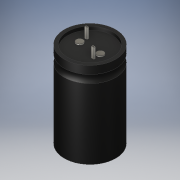
# Autodesk Inventor part: capacitor (LGN2X151MELB50)
Saved by Autodesk Inventor 2017 (Build 210142000, 142)
## iProperties
Part Number: capacitor (LGN2X151MELB50)
Material: Generisch
Document SubType Name: Modeling
Designer: ExCISS
Density: 1 g/cm^3
Appearance: Glänzend - schwarz
Author: ExCISS
Autodesk Inventor part; units mm, degrees
ref_plane "YZ Plane" through (0, 0, 0) normal (1, 0, 0) x (0, 1, 0)
ref_plane "XZ Plane" through (0, 0, 0) normal (0, 1, 0) x (-1, 0, 0)
sketch "Skizze1" plane through (0, 0, 0) normal (0, 1, 0) x (-1, 0, 0)
  line L0 (0, 0) -> (0, 50)
  line L1 (0, 50) -> (-15, 50)
  line L2 (-15, 50) -> (-15, 45.4)
  line L3 (-15, 40.8) -> (-15, 0)
  arc A0 (-15, 40.8) -> (-15, 45.4) centre (-20.6528, 43.1) ccw
  line L4 (0, 0) -> (-15, 0)
  line L5 (0, -10) -> (0, 60) projected
  dimension "d0" = 50
  dimension "d1" = 15
  dimension "d2" = 4.6
  dimension "d72" = 14.55
  dimension "d73" = 4.6
  constraints: 10 end point, 2 perpendicular, 2 point on circle, 2 point on line, 1 centre point, 1 horizontal, 1 vertical
  measures "d0" distance of L0.start L0.end
  measures "d1" distance of L0.end L1.end
  measures "d2" distance of L1.end L2.end
  measures "d72" distance edge to line of A0 L0
  measures "d73" distance of L2.end L3.start
revolve "Umdrehung1" add sketch "Skizze1" angle 360 about axis through (0, 0, -10) along (0, 0, 1)
sketch "Skizze3" plane through (0, 0, 50) normal (0, 0, 1) x (1, 0, 0)
  circle A0 centre (0, 0) radius 13.05
  dimension "d10" = 26.1
  constraints: 1 centre point, 1 coincident
  measures "d10" diameter of A0
extrude "Extrusion2" cut sketch "Skizze3" against normal blind 2
sketch "Skizze7" plane through (0, 0, 0) normal (0, 0, -1) x (-1, 0, 0)
  circle A0 centre (0, 0) radius 12.8
  dimension "d19" = 25.6
  constraints: 1 centre point, 1 coincident
  measures "d19" diameter of A0
extrude "Extrusion4" cut sketch "Skizze7" against normal blind 0.02
sketch "Skizze17" plane through (0, 0, 48) normal (0, 0, 1) x (1, 0, 0)
  line L0 (-4.2414, 0) -> (6, 0) construction
  line L1 (6, 0) -> (-6, 0) construction
  line L2 (6, 0) -> (6, -3.5) construction
  line L3 (-6, 0) -> (-6, 3.5) construction
  line L4 (-6, 3.5) -> (6, -3.5) construction
  circle A0 centre (-6, 0) radius 2
  circle A1 centre (6, 0) radius 2
  line L5 (-6.75, 4.5) -> (-5.25, 4.5)
  line L6 (-5.25, 4.5) -> (-5.25, 3.5)
  line L7 (-5.25, 3.5) -> (-6.75, 3.5)
  line L8 (-6.75, 3.5) -> (-6.75, 4.5)
  line L9 (6.75, -3.5) -> (5.25, -3.5)
  line L10 (5.25, -3.5) -> (5.25, -4.5)
  line L11 (5.25, -4.5) -> (6.75, -4.5)
  line L12 (6.75, -4.5) -> (6.75, -3.5)
  point P0 (0, 0)
  point P1 (0, 0)
  dimension "d54" = 12
  dimension "d55" = 3.5
  dimension "d56" = 3.5
  dimension "d57" = 4
  dimension "d58" = 4
  dimension "d59" = 1.5
  dimension "d60" = 1
  dimension "d61" = 1.5
  dimension "d62" = 1
  constraints: 26 end point, 4 parallel, 3 coincident, 3 horizontal, 3 midpoint, 2 centre point, 2 perpendicular, 2 vertical, 1 point on line
  measures "d54" distance of L0.end L1.end
  measures "d55" distance of L2.end L0.end
  measures "d56" distance of L3.end L1.end
  measures "d57" diameter of A0
  measures "d58" diameter of A1
  measures "d59" distance of L6.end L7.end
  measures "d60" distance of L5.end L6.end
  measures "d61" distance of L11.end L10.end
  measures "d62" distance of L10.end L9.end
extrude "Extrusion8" add sketch "Skizze17" along normal blind 0.6 contours A0 | A1
sketch "Skizze18" plane through (0, 0, 48) normal (0, 0, 1) x (1, 0, 0)
  line L0 (-6.75, 4.5) -> (-5.25, 4.5)
  line L1 (-5.25, 4.5) -> (-5.25, 3.5)
  line L2 (-5.25, 3.5) -> (-6.75, 3.5)
  line L3 (-6.75, 3.5) -> (-6.75, 4.5)
  line L4 (6.75, -3.5) -> (5.25, -3.5)
  line L5 (5.25, -3.5) -> (5.25, -4.5)
  line L6 (5.25, -4.5) -> (6.75, -4.5)
  line L7 (6.75, -4.5) -> (6.75, -3.5)
  point P0 (0, 0)
  point P1 (-6, 3.5)
  point P2 (6, -3.5)
  dimension "d66" = 1.5
  dimension "d67" = 1
  dimension "d68" = 1.5
  dimension "d69" = 1
  constraints: 16 end point, 4 parallel, 2 horizontal, 2 midpoint, 2 perpendicular
  measures "d66" distance of L1.end L2.end
  measures "d67" distance of L1.start L1.end
  measures "d68" distance of L6.end L5.end
  measures "d69" distance of L5.end L4.end
extrude "Extrusion9" add sketch "Skizze18" along normal blind 6
sketch "Skizze9" plane through (0, 0, 0.02) normal (0, 0, -1) x (-1, 0, 0)
  line L0 (-7.5, 0) -> (7.5, 0) construction
  line L1 (0, 4.0384) -> (0, 7.5) construction
  line L2 (0, 7.5) -> (0, -7.5) construction
  line L3 (0.15, 7.5) -> (-0.15, 7.5)
  line L4 (-0.15, 7.5) -> (-0.15, 0.15)
  line L5 (-0.15, 0.15) -> (-7.5, 0.15)
  line L6 (-7.5, 0.15) -> (-7.5, -0.15)
  line L7 (-7.5, -0.15) -> (-0.15, -0.15)
  line L8 (-0.15, -0.15) -> (-0.15, -7.5)
  line L9 (-0.15, -7.5) -> (0.15, -7.5)
  line L10 (0.15, -7.5) -> (0.15, -0.15)
  line L11 (0.15, -0.15) -> (7.5, -0.15)
  line L12 (7.5, -0.15) -> (7.5, 0.15)
  line L13 (7.5, 0.15) -> (0.15, 0.15)
  line L14 (0.15, 0.15) -> (0.15, 7.5)
  point P0 (0, 0)
  point P1 (0, 0)
  dimension "d23" = 15
  dimension "d24" = 15
  dimension "d74" = 0.3
  constraints: 30 end point, 12 perpendicular, 6 midpoint, 4 equal length, 1 coincident, 1 horizontal, 1 point on line
  measures "d23" distance of L0.start L0.end
  measures "d24" distance of L1.end L2.end
  measures "d74" distance between parallel lines of L10 L8
extrude "Extrusion10" cut sketch "Skizze9" against normal blind 0.3
sketch "Skizze19" plane through (0, 0, 54) normal (0, 0, 1) x (1, 0, 0)
  line L0 (6.75, -3.5) -> (5.25, -3.5) projected
  line L1 (6.75, -3.5) -> (5.25, -3.5) projected
  line L2 (5.25, -3.5) -> (5.25, -4.5) projected
  line L3 (5.25, -4.5) -> (6.75, -4.5) projected
  line L4 (6.75, -4.5) -> (6.75, -3.5) projected
  line L5 (5.25, -3.5) -> (6.75, -4.5) construction
  circle A0 centre (6, -4) radius 0.25
  line L6 (-5.25, 3.5) -> (-5.25, 4.5) projected
  line L7 (-5.25, 4.5) -> (-6.75, 4.5) projected
  line L8 (-6.75, 4.5) -> (-6.75, 3.5) projected
  line L9 (-6.75, 3.5) -> (-5.25, 3.5) projected
  line L10 (-5.25, 4.5) -> (-6.75, 4.5) construction
  line L11 (-6.75, 4.5) -> (-5.25, 3.5) construction
  circle A1 centre (-6, 4) radius 0.25
  point P0 (0, 0)
  dimension "d77" = 0.5
  dimension "d78" = 0.5
  constraints: 4 end point, 2 centre point, 2 midpoint
  measures "d77" diameter of A0
  measures "d78" diameter of A1
extrude "Extrusion11" add sketch "Skizze19" along normal blind 0.001 contours A0 | A1
ref_plane "Arbeitsebene1" through (-6, 4, 54.001) normal (0.5547, 0.8321, 0) x (0, 0, 1)
